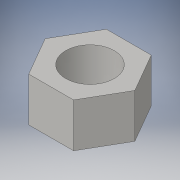
# Autodesk Inventor part: 3-8 Inch Hex Nut
Saved by Autodesk Inventor 2016 (Build 200138000, 138)
## iProperties
Created: 2016-01-28
Part Number: 3-8 Inch Hex Nut
Material: Generic
Document SubType Name: Modeling
Designer: Jack Jaworski
Density: 1 g/cm^3
Appearance: Default
Author: Jack Jaworski
Autodesk Inventor part; units mm, degrees
ref_plane "YZ Plane" through (0, 0, 0) normal (1, 0, 0) x (0, 1, 0)
ref_plane "XZ Plane" through (0, 0, 0) normal (0, 1, 0) x (-1, 0, 0)
ref_plane "XY Plane" through (0, 0, 0) normal (0, 0, 1) x (1, 0, 0)
sketch "Sketch1" plane through (0, 0, 0) normal (0, 1, 0) x (-1, 0, 0)
  line L0 (4.3994, -7.62) -> (-4.3994, -7.62)
  line L1 (-4.3994, -7.62) -> (-8.7988, 0)
  line L2 (-8.7988, 0) -> (-4.3994, 7.62)
  line L3 (-4.3994, 7.62) -> (4.3994, 7.62)
  line L4 (4.3994, 7.62) -> (8.7988, 0)
  line L5 (8.7988, 0) -> (4.3994, -7.62)
  circle A0 centre (0, 0) radius 4.7625
  dimension "d0" = 15.24
  dimension "d1" = 9.525
  constraints: 12 end point, 2 coincident, 1 centre point, 1 horizontal, 13 other
  measures "d0" distance between parallel lines of L0 L3
  measures "d1" diameter of A0
extrude "Extrusion1" add sketch "Sketch1" along normal blind 8.636
body "Solid1"
